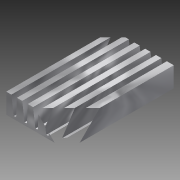
# Autodesk Inventor part: HeatSink60
Saved by Autodesk Inventor 2014 (Build 180170000, 170)
## iProperties
Created: 2015-04-18
Part Number: HeatSink60
Material: Generic
Document SubType Name: Modeling
Designer: Owner
Density: 1 g/cm^3
Appearance: Aluminum - Polished
Author: Owner
Autodesk Inventor part; units mm, degrees
ref_plane "YZ Plane" through (0, 0, 0) normal (1, 0, 0) x (0, 1, 0)
ref_plane "XZ Plane" through (0, 0, 0) normal (0, 1, 0) x (-1, 0, 0)
ref_plane "XY Plane" through (0, 0, 0) normal (0, 0, 1) x (1, 0, 0)
sketch "Sketch1" plane through (0, 0, 0) normal (0, 1, 0) x (-1, 0, 0)
  line L0 (-3.1407, 29.7008) -> (54.0093, 29.7008)
  line L1 (54.0093, 29.7008) -> (54.0093, -70.2992)
  line L2 (54.0093, -70.2992) -> (-3.1407, -70.2992)
  line L3 (-3.1407, -70.2992) -> (-3.1407, 29.7008)
  point P0 (0, 0)
  dimension "d0" = 57.15
  dimension "d1" = 100
  constraints: 8 end point, 2 parallel, 1 horizontal, 1 perpendicular
  measures "d0" distance of L0.start L0.end
  measures "d1" distance of L0.end L1.end
extrude "Extrusion1" add sketch "Sketch1" along normal blind 18.8
sketch "Sketch3" plane through (-54.0093, 0, 29.7008) normal (0, 0, 1) x (1, 0, 0)
  line L0 (0, 18.8) -> (57.15, 18.8)
  line L1 (2.6537, 35.2563) -> (7.0386, 2.4572)
  line L2 (7.0386, 2.4572) -> (9.3017, 2.7597)
  line L3 (9.3017, 2.7597) -> (10.7219, 35.2563)
  line L4 (10.7219, 35.2563) -> (2.6537, 35.2563)
  point P0 (54.0093, 0)
  point P1 (29.7008, 0)
  constraints: 10 end point, 1 parallel, 1 perpendicular
extrude "Extrusion3" cut sketch "Sketch3" against normal through all
pattern_linear "Rectangular Pattern1" count 5 spacing 10.16 along (1, 0, 0) of "Extrusion3"
sketch "Sketch4" plane through (0, 18.8, 0) normal (0, 1, 0) x (1, 0, 0)
  point P0 (-0.0093, -5.7008)
hole "Hole1" at (-0.0093, 18.8, 5.7008) direction (0, -1, 0) diameter 3.4544 depth 18.8
sketch "Sketch5" plane through (0, 18.8, 0) normal (0, 1, 0) x (1, 0, 0)
  point P0 (-52.0093, -5.7008)
hole "Hole3" at (-52.0093, 18.8, 5.7008) direction (0, -1, 0) diameter 3.4544 depth 18.8
sketch "Sketch6" plane through (0, 18.8, 0) normal (0, 1, 0) x (1, 0, 0)
  point P0 (-0.0093, 46.2992)
hole "Hole5" at (-0.0093, 18.8, -46.2992) direction (0, -1, 0) diameter 3.4544 depth 18.8
sketch "Sketch7" plane through (0, 18.8, 0) normal (0, 1, 0) x (1, 0, 0)
  point P0 (-52.0093, 46.2992)
hole "Hole7" at (-52.0093, 18.8, -46.2992) direction (0, -1, 0) diameter 3.4544 depth 18.8
body "Solid1"
